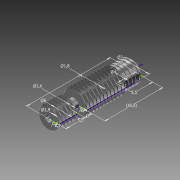
# Autodesk Inventor part: Heat Break
Saved by Autodesk Inventor 2015 (Build 190159000, 159)
## iProperties
Created: 2015-02-05
Part Number: Heat Break
Material: Типовые
Document SubType Name: Modeling
Designer: Parabolik
Density: 1 g/cm^3
Appearance: Сталь — полированная
Author: Parabolik
Autodesk Inventor part; units mm, degrees
ref_plane "YZ Plane" through (0, 0, 0) normal (1, 0, 0) x (0, 1, 0)
ref_plane "XZ Plane" through (0, 0, 0) normal (0, 1, 0) x (-1, 0, 0)
ref_plane "XY Plane" through (0, 0, 0) normal (0, 0, 1) x (1, 0, 0)
sketch "Эскиз1" plane through (0, 0, 0) normal (0, 0, 1) x (1, 0, 0)
  line L0 (0, 0) -> (0, 27)
  line L1 (0.95, 0) -> (3, 0)
  line L2 (3, 0) -> (3, 5.5)
  line L3 (3, 5.5) -> (1.3, 5.5)
  line L4 (1.3, 5.5) -> (1.3, 7.5)
  line L5 (1.3, 7.5) -> (3.5, 7.5)
  line L6 (3.5, 7.5) -> (3.5, 24)
  line L7 (3.5, 24) -> (2, 24)
  line L8 (0.9, 18.5) -> (0.9, 7.5)
  line L9 (0.95, 0) -> (0.95, 5.5)
  line L10 (0.9, 7.5) -> (0.95, 5.5)
  line L11 (2, 24) -> (2, 19)
  line L12 (2, 19) -> (0.9, 18.5)
  line L13 (3.5, 7.5) -> (3.5, 6.6)
  line L14 (3, 0) -> (3, -0.9)
  line L15 (3, -0.9) -> (3, -0.45)
  line L16 (3, 7.1) -> (3.5, 7.5)
  line L17 (2.5, -0.4) -> (3, 0)
  line L18 (3, 7.1) -> (3, 7)
  line L19 (3, 7) -> (3.5, 6.6)
  line L20 (2.5, -0.4) -> (2.5, -0.5)
  line L21 (2.5, -0.5) -> (3, -0.9)
  dimension "d3" = 2
  dimension "d4" = 7
  dimension "d5" = 24
  dimension "d6" = 2.6
  dimension "d7" = 6
  dimension "d10" = 1.8
  dimension "d12" = 1.9
  dimension "d13" = 5.5
  dimension "d14" = 5
  dimension "d15" = 4
  dimension "d16" = 5.5
  dimension "d30" = 16.5
  dimension "d40" = 0.9
  dimension "d52" = 0.9
  dimension "d56" = 0.1
  dimension "d57" = 0.1
  constraints: 44 end point, 7 vertical, 6 perpendicular, 1 horizontal, 1 midpoint, 1 parallel
  measures "d3" distance of L3.end L4.end
  measures "d4" diameter of L6 L0
  measures "d5" distance between parallel lines of L7 L1
  measures "d6" diameter of L4 L0
  measures "d7" diameter of L2 L0
  measures "d10" diameter of L8 L0
  measures "d12" diameter of L9 L0
  measures "d13" distance from line of L8.start L7
  measures "d14" distance of L7.end L11.end
  measures "d15" diameter of L11 L0
  measures "d16" distance between parallel lines of L3 L1
  measures "d30" distance between parallel lines of L7 L5
  measures "d40" distance of L5.end L13.end
  measures "d52" distance of L1.end L14.end
  measures "d56" distance of L16.start L18.end
  measures "d57" distance of L17.start L20.end
revolve "Вращение1" add sketch "Эскиз1" angle 360 about axis through (0, 0, 0) along (0, 1, 0) contours L9 L10 L8 L12 L11 L7 L6 L5 L4 L3 L2 L1
thread "Резьба1" size "M6x1" class "6g" standard "ANSI Metric M Profile" full length
coil "Пружина1" sketch "Эскиз1" operation cut axis through (0, 0, 0) along (0, 1, 0) pitch 1 turns 6.5 hand right contours L14 L21 L20 L17
thread "Резьба2" size "M7x1" class "6g" standard "ANSI Metric M Profile" full length
coil "Пружина2" sketch "Эскиз1" operation cut axis through (0, 0, 0) along (0, 1, 0) pitch 1 turns 16.5 hand right contours L13 L19 L18 L16
sketch "Эскиз2" plane through (0, 24, 0) normal (0, 1, 0) x (1, 0, 0)
  circle A0 centre (0, 0) radius 0.9 projected
  circle A1 centre (0, 0) radius 3.1
  circle A2 centre (0, 0) radius 3.5
  dimension "d23" = 6.2
  dimension "d29" = 7
  constraints: 2 centre point, 1 coincident
  measures "d23" diameter of A1
  measures "d29" diameter of A2
extrude "Выдавливание1" cut sketch "Эскиз2" against normal blind 5 contours A2
chamfer "Фаска1" distance 0.5 angle 45 1 edges at (-3.1, 24, 0)
